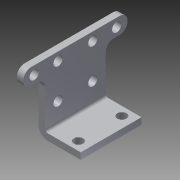
# Autodesk Inventor part: M - Hook Mount Bracket
Saved by Autodesk Inventor 2013 (Build 170138000, 138)
## iProperties
Created: 2013-02-20
Part Number: M - Hook Mount Bracket
Material: Aluminum 6061
Document SubType Name: Sheet Metal
Designer: Moses
Mass: 45.3805 g
Surface Area: 92.6426 cm^2
Volume: 16.7456 cm^3
Density: 2.71 g/cm^3
Sheet Metal Rule: Default
Author: Moses
Autodesk Inventor part; units mm, degrees
ref_plane "YZ Plane" through (0, 0, 0) normal (1, 0, 0) x (0, 1, 0)
ref_plane "XZ Plane" through (0, 0, 0) normal (0, 1, 0) x (-1, 0, 0)
ref_plane "XY Plane" through (0, 0, 0) normal (0, 0, 1) x (1, 0, 0)
sketch "Sketch1" plane through (0, 0, 0) normal (0, 1, 0) x (-1, 0, 0)
  line L0 (0, 0) -> (35.56, 0)
  line L1 (35.56, 0) -> (35.56, 44.45)
  line L2 (35.56, 44.45) -> (0, 44.45)
  line L3 (0, 44.45) -> (0, 0)
  line L4 (12.7, 38.1) -> (12.7, 6.35) construction
  circle A0 centre (12.7, 38.1) radius 3.3782
  circle A1 centre (12.7, 6.35) radius 3.3782
  line L5 (0, 22.225) -> (35.56, 22.225) construction
  point P0 (12.7, 22.225)
  dimension "d0" = 35.56
  dimension "d2" = 44.45
  dimension "d3" = 6.7564
  dimension "d4" = 31.75
  dimension "d16" = 12.7
  measures "d0" distance of L1.end L2.end
  measures "d2" distance of L0.end L1.end
  measures "d3" diameter of A0
  measures "d4" distance of L4.start L4.end
  measures "d16" distance between parallel lines of L4 L3
extrude "Plate1" add sketch "Sketch1" along normal blind 4.7625
sketch "Sketch2" plane through (-30.7975, 0, 44.45) normal (-1, 0, 0) x (0, -1, 0)
  line L0 (0, -44.45) -> (0, 0)
  line L1 (0, 0) -> (-50.8, 0)
  line L2 (-50.8, 0) -> (-50.8, -44.45)
  line L3 (-50.8, -44.45) -> (0, -44.45)
  constraints: 6 end point, 1 horizontal, 1 perpendicular, 1 vertical
edge flange "Flange1" height 50.8 angle 90 thickness 4.7625 bend radius 1.905 thickness toward (-1, 0, 0) relief straight relief width 4.7625 relief depth 2.3813 edges at (-35.56, 4.7625, 22.225) wall of the first edge with corners at (-30.7975, 0, 0) (-30.7975, 0, 44.45) (-30.7975, 50.8, 44.45) (-30.7975, 50.8, 0)
bend "Bend1"
corner "Corner1"
sketch "Sketch3" plane through (-35.56, 50.8, 0) normal (-1, 0, 0) x (0, 0, 1)
  line L0 (0, -44.1325) -> (44.45, -44.1325) projected
  line L1 (0, 0) -> (44.45, 0) projected
  line L2 (0, -44.1325) -> (0, 0) projected
  circle A0 centre (9.525, -6.0325) radius 3.3782
  circle A1 centre (34.925, -6.0325) radius 3.3782
  line L3 (9.525, -6.0325) -> (34.925, -6.0325) construction
  line L4 (22.225, 0) -> (22.225, -44.1325) construction
  line L5 (44.45, 0) -> (44.45, -44.1325) projected
  circle A2 centre (9.525, -31.4325) radius 3.3782
  line L6 (9.525, -31.4325) -> (34.925, -31.4325) construction
  circle A3 centre (34.925, -31.4325) radius 3.3782
  line L7 (44.45, -12.065) -> (60.325, -12.065)
  line L8 (60.325, -12.065) -> (60.325, 0)
  line L9 (60.325, 0) -> (44.45, 0)
  line L10 (0, -12.065) -> (-15.875, -12.065)
  line L11 (-15.875, -12.065) -> (-15.875, 0)
  line L12 (-15.875, 0) -> (0, 0)
  circle A4 centre (-7.9375, -6.0325) radius 3.3782
  circle A5 centre (52.3875, -6.0325) radius 3.3782
  line L13 (-7.9375, 0) -> (-7.9375, -12.065) construction
  line L14 (52.3875, -12.065) -> (52.3875, 0) construction
  line L15 (-7.9375, -6.0325) -> (52.3875, -6.0325) construction
  point P0 (0, -50.8)
  point P1 (22.225, -6.0325)
  point P2 (22.225, -31.4325)
  dimension "d18" = 6.7564
  dimension "d19" = 38.1
  dimension "d20" = 25.4
  dimension "d23" = 25.4
  dimension "d24" = 6.7564
  dimension "d25" = 25.4
  dimension "d26" = 15.875
  dimension "d27" = 15.875
  dimension "d28" = 12.065
  dimension "d29" = 12.065
  dimension "d35" = 6.7564
  dimension "d42" = 6.0325
  constraints: 24 end point, 11 midpoint, 6 centre point, 5 perpendicular, 4 point on line, 3 equal radius, 3 parallel, 1 coincident, 1 collinear
  measures "d18" diameter of A1
  measures "d19" distance between parallel lines of L0 L3
  measures "d20" distance of L3.start L3.end
  measures "d23" distance of L6.start L6.end
  measures "d24" diameter of A3
  measures "d25" distance between parallel lines of L6 L3
  measures "d26" distance of L11.end L1.start
  measures "d27" distance of L8.end L1.end
  measures "d28" distance of L7.end L8.end
  measures "d29" distance of L10.end L11.end
  measures "d35" diameter of A4
  measures "d42" distance from line of L1 L3.start
sheet face with bend "Face2" sketch "Sketch3" thickness 4.7625 toward (1, 0, 0) bend radius 4.7625 relief straight relief width 4.7625 relief depth 2.3813 contours L10 L11 L12 L2 | L5 L9 L8 L7 | A4 | A5
bend "Bend2"
extrude "Cut2" cut sketch "Sketch3" against normal blind 4.7625 contours A0 | A1 | A2 | A3 | A4 | A5
fillet "Corner Round1" radius 5.715 6 edges at (-33.1788, 38.735, 44.45) (-33.1788, 38.735, 0) (-33.1788, 50.8, -15.875) (-33.1788, 38.735, -15.875) (-33.1788, 38.735, 60.325) (-33.1788, 50.8, 60.325)
sketch "Sketch4" plane through (0, 0, 0) normal (0, -1, 0) x (1, 0, 0)
  line L0 (0, 0) -> (-28.8925, 0) projected
  line L1 (0, 44.45) -> (0, 0) projected
  line L2 (-28.8925, 44.45) -> (0, 44.45) projected
  line L3 (-4.699, 44.45) -> (-4.699, 0)
  dimension "d39" = 4.699
  constraints: 2 end point, 2 point on line, 1 perpendicular
  measures "d39" distance between parallel lines of L1 L3
extrude "Cut3" cut sketch "Sketch4" against normal blind 4.7625
equation "\"d27\" = d26"
equation "\"d28\" = 2 * d42"
equation "\"d29\" = d28"
equation "\"d35\" = d18"
equation "\"d36\" = Thickness"
equation "\"d40\" = Thickness"
equation "\"d6\" = BendReliefWidth"
equation "\"d7\" = BendReliefDepth"
equation "\"d8\" = MinimumRemnant"
equation "\"d9\" = BendRadius"
equation "\"d13\" = CornerReliefSize"
equation "\"d14\" = GapSize"
equation "\"d15\" = JacobiRadiusSize"
equation "\"d30\" = BendRadius"
equation "\"d31\" = BendReliefWidth"
equation "\"d33\" = MinimumRemnant"
equation "\"d32\" = BendReliefDepth"
equation "\"d34\" = BendRadius"
equation "\"BendRadius\" = Thickness"
equation "\"BendReliefWidth\" = Thickness"
equation "\"BendReliefDepth\" = 0.5 * Thickness"
equation "\"CornerReliefSize\" = 4 * Thickness"
equation "\"MinimumRemnant\" = 2 * Thickness"
equation "\"TransitionRadius\" = BendRadius"
equation "\"JacobiRadiusSize\" = BendRadius"
equation "\"GapSize\" = Thickness"
equation "\"d5\" = BendRadius"
equation "\"Thickness\" = 4.7625"
body "Solid1"
